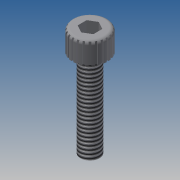
# Autodesk Inventor part: screw_10
Saved by Autodesk Inventor 2014 SP1 (Build 180222100, 222)
## iProperties
Created: 2014-08-29
Part Number: screw_10
Material: Generic
Document SubType Name: Modeling
Designer: Dave
Density: 1 g/cm^3
Appearance: Default
Author: Dave
Autodesk Inventor part; units mm, degrees
ref_plane "YZ Plane" through (0, 0, 0) normal (1, 0, 0) x (0, 1, 0)
ref_plane "XZ Plane" through (0, 0, 0) normal (0, 1, 0) x (-1, 0, 0)
ref_plane "XY Plane" through (0, 0, 0) normal (0, 0, 1) x (1, 0, 0)
sketch "Sketch1" plane through (0, 0, 0) normal (0, 1, 0) x (-1, 0, 0)
  circle A0 centre (0, 0) radius 3.81
  dimension "d0" = 7.62
  constraints: 1 centre point, 1 coincident
  measures "d0" diameter of A0
extrude "Extrusion1" add sketch "Sketch1" along normal blind 4.572
sketch "Sketch2" plane through (0, 4.572, 0) normal (0, 1, 0) x (1, 0, 0)
  circle A0 centre (0, 0) radius 3.81 projected
  line L0 (1.6912, -0.9423) -> (0.0296, -1.9358)
  line L1 (0.0296, -1.9358) -> (-1.6616, -0.9935)
  line L2 (-1.6616, -0.9935) -> (-1.6912, 0.9423)
  line L3 (-1.6912, 0.9423) -> (-0.0296, 1.9358)
  line L4 (-0.0296, 1.9358) -> (1.6616, 0.9935)
  line L5 (1.6616, 0.9935) -> (1.6912, -0.9423)
  constraints: 12 end point, 1 coincident, 13 other
extrude "Extrusion2" cut sketch "Sketch2" against normal blind 2.54 contours L0 L1 L2 L3 L4 L5
fillet "Fillet1" radius 0.762 1 edges at (3.81, 4.572, 0)
sketch "Sketch3" plane through (0, 0, 0) normal (0, -1, 0) x (1, 0, 0)
  circle A0 centre (0, 0) radius 3.81 projected
  circle A1 centre (0, 0) radius 2.0574
  dimension "d6" = 4.1148
  constraints: 1 centre point, 1 coincident
  measures "d6" diameter of A1
extrude "Extrusion3" add sketch "Sketch3" along normal blind 19.05 contours A1
thread "Thread3" size "8-32 UNC" class "2A" standard "ANSI Unified Screw Threads" full length
sketch "Sketch4" plane through (0, 0, 0) normal (0, -1, 0) x (1, 0, 0)
  circle A0 centre (0, 0) radius 2.0574 projected
  circle A1 centre (0, 0) radius 3.81 projected
  point P0 (0, 3.81)
  constraints: 1 vertical alignment, 1 other
ref_plane "Work Plane1" through (0, 0, 3.81) normal (0, 0, 1) x (1, 0, 0)
sketch "Sketch5" plane through (0, 0, 3.81) normal (0, 0, 1) x (1, 0, 0)
  line L0 (-0.1969, 0) -> (0.1841, 0)
  line L1 (0.1841, 0) -> (0.1841, 4.8075)
  line L2 (0.1841, 4.8075) -> (-0.1969, 4.8075)
  line L3 (-0.1969, 4.8075) -> (-0.1969, 0)
  point P0 (0, 0)
  dimension "d15" = 0.381
  constraints: 8 end point, 2 parallel, 1 horizontal, 1 perpendicular
  measures "d15" distance of L2.end L1.end
extrude "Extrusion4" cut sketch "Sketch5" against normal blind 0.254
pattern_circular "Circular Pattern1" count 24 over 360 about axis through (0, 0, 0) along (0, -1, 0) of "Extrusion4"
body "Solid1"
